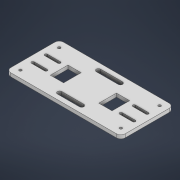
# Autodesk Inventor part: Top
Saved by Autodesk Inventor 2022.1 (Build 261234000, 234)
## iProperties
Created: 2021-10-08
Part Number: Top
Material: Generic
Document SubType Name: Modeling
Designer: Santiago Martínez
Mass: 26.6109 g
Surface Area: 166.584 cm^2
Volume: 26.6109 cm^3
Density: 1 g/cm^3
Appearance: Default
Author: Santiago Martínez
Autodesk Inventor part; units mm, degrees
ref_plane "YZ Plane" through (0, 0, 0) normal (1, 0, 0) x (0, 1, 0)
ref_plane "XZ Plane" through (0, 0, 0) normal (0, 1, 0) x (-1, 0, 0)
ref_plane "XY Plane" through (0, 0, 0) normal (0, 0, 1) x (1, 0, 0)
sketch "Motor Support" plane through (0, 0, 0) normal (1, 0, 0) x (0, 1, 0)
  circle A0 centre (0, 0) radius 11.25
  line L0 (-12.5, -22.5) -> (22.5, -22.5)
  line L1 (22.5, -22.5) -> (22.5, 22.5)
  line L2 (22.5, 22.5) -> (-12.5, 22.5)
  line L3 (-22.5, 12.5) -> (-22.5, -12.5)
  arc A1 (-12.5, 22.5) -> (-22.5, 12.5) centre (-12.5, 12.5) ccw
  arc A2 (-22.5, -12.5) -> (-12.5, -22.5) centre (-12.5, -12.5) ccw
  circle A3 centre (15.5, 15.5) radius 1.5
  circle A4 centre (15.5, -15.5) radius 1.5
  circle A5 centre (-15.5, 15.5) radius 1.5
  circle A6 centre (-15.5, -15.5) radius 1.5
  point P0 (-22.5, 22.5)
  point P1 (22.5, 0)
  dimension "d0" = 22.5
  dimension "d1" = 45
  dimension "d2" = 45
  dimension "d3" = 10
  dimension "d4" = 22.5
  dimension "d5" = 3
  dimension "d6" = 3
  dimension "d7" = 3
  dimension "d8" = 3
  dimension "d9" = 31
  dimension "d10" = 31
  dimension "d11" = 15.5
  dimension "d12" = 15.5
  constraints: 8 end point, 7 centre point, 4 point on circle, 4 tangent, 3 horizontal alignment, 2 parallel, 2 point on line, 2 vertical alignment, 1 coincident, 1 equal radius, 1 horizontal, 1 midpoint, 1 perpendicular
  measures "d0" diameter of A0
  measures "d1" distance of point (-22.5, 22.5) L1.end
  measures "d2" distance of L1.end L0.end
  measures "d3" radius of A1
  measures "d4" distance from line of L1 point (0, 0)
  measures "d5" diameter of A3
  measures "d6" diameter of A4
  measures "d7" diameter of A5
  measures "d8" diameter of A6
  measures "d9" distance of A4.centre A3.centre
  measures "d10" distance of A5.centre A3.centre
  measures "d11" horizontal distance of A3.centre point (0, 0)
  measures "d12" horizontal distance of A3.centre point (0, 0)
extrude "Motor Support E" add sketch "Motor Support" along normal blind 4
sketch "Base" plane through (0, 22.5, 22.5) normal (0, 1, 0) x (1, 0, 0)
  line L0 (0, 45) -> (0, 0) projected
  line L1 (0, 0) -> (4, 0) projected
  line L2 (4, 45) -> (4, 0) projected
  line L3 (0, 45) -> (4, 45) projected
  line L4 (4, -7.5) -> (-61, -7.5)
  line L5 (-61, -7.5) -> (-61, 52.5)
  line L6 (-61, 52.5) -> (4, 52.5)
  line L7 (4, 52.5) -> (4, -7.5)
  line L8 (-41, 32.5) -> (-26, 32.5)
  line L9 (-26, 32.5) -> (-26, 12.5)
  line L10 (-26, 12.5) -> (-41, 12.5)
  line L11 (-41, 12.5) -> (-41, 32.5)
  point P0 (0, 22.5)
  point P1 (4, 22.5)
  point P2 (-26, 22.5)
  point P3 (0, 22.5)
  dimension "d15" = 65
  dimension "d16" = 60
  dimension "d19" = 15
  dimension "d20" = 20
  dimension "d21" = 26
  constraints: 16 end point, 4 midpoint, 4 parallel, 2 horizontal, 2 perpendicular, 1 horizontal alignment
  measures "d15" distance of L5.end L6.end
  measures "d16" distance of L4.end L5.end
  measures "d19" distance of L9.end L10.end
  measures "d20" distance of L8.end L9.end
  measures "d21" distance between parallel lines of L0 L9
extrude "Base E" add sketch "Base" along normal blind 4
ref_plane "Mid Plane" through (-61, 26.5, 30) normal (-1, 0, 0) x (0, 0, 1)
mirror "Mirror Base" about plane through (-61, 26.5, 30) normal (-1, 0, 0)
fillet "Fillet1" radius 5 4 edges at (4, 24.5, 30) (4, 24.5, -30) (-126, 24.5, 30) (-126, 24.5, -30)
sketch "Base Hole Pattern" plane through (0, 26.5, 22.5) normal (0, 1, 0) x (1, 0, 0)
  circle A0 centre (-4, 0.5) radius 1.5
  circle A1 centre (-118, 44.5) radius 1.5
  circle A2 centre (-118, 0.5) radius 1.5
  circle A3 centre (-4, 44.5) radius 1.5
  arc A4 (-121, 52.5) -> (-126, 47.5) centre (-121, 47.5) ccw projected
  line L0 (-126, -2.5) -> (-126, 47.5) projected
  arc A5 (-126, -2.5) -> (-121, -7.5) centre (-121, -2.5) ccw projected
  line L1 (-1, -7.5) -> (-121, -7.5) projected
  arc A6 (-1, -7.5) -> (4, -2.5) centre (-1, -2.5) ccw projected
  line L2 (4, -2.5) -> (4, 47.5) projected
  arc A7 (4, 47.5) -> (-1, 52.5) centre (-1, 47.5) ccw projected
  line L3 (-1, 52.5) -> (-121, 52.5) projected
  line L4 (-81, 32.5) -> (-96, 32.5) projected
  line L5 (-81, 12.5) -> (-81, 32.5) projected
  line L6 (-96, 12.5) -> (-81, 12.5) projected
  line L7 (-96, 32.5) -> (-96, 12.5) projected
  line L8 (-41, 32.5) -> (-26, 32.5) projected
  line L9 (-26, 32.5) -> (-26, 12.5) projected
  line L10 (-26, 12.5) -> (-41, 12.5) projected
  line L11 (-41, 12.5) -> (-41, 32.5) projected
  line L12 (-73.5, 44.5) -> (-48.5, 44.5) construction
  line L13 (-73.5, 42) -> (-48.5, 42)
  line L14 (-48.5, 47) -> (-73.5, 47)
  arc A8 (-73.5, 47) -> (-73.5, 42) centre (-73.5, 44.5) ccw
  arc A9 (-48.5, 42) -> (-48.5, 47) centre (-48.5, 44.5) ccw
  line L15 (-73.5, 0.5) -> (-48.5, 0.5) construction
  line L16 (-73.5, -2) -> (-48.5, -2)
  line L17 (-48.5, 3) -> (-73.5, 3)
  arc A10 (-73.5, 3) -> (-73.5, -2) centre (-73.5, 0.5) ccw
  arc A11 (-48.5, -2) -> (-48.5, 3) centre (-48.5, 0.5) ccw
  line L18 (-118.5, 30) -> (-103.5, 30) construction
  line L19 (-118.5, 28.5) -> (-103.5, 28.5)
  line L20 (-103.5, 31.5) -> (-118.5, 31.5)
  arc A12 (-118.5, 31.5) -> (-118.5, 28.5) centre (-118.5, 30) ccw
  arc A13 (-103.5, 28.5) -> (-103.5, 31.5) centre (-103.5, 30) ccw
  line L21 (-118.5, 15) -> (-103.5, 15) construction
  line L22 (-118.5, 13.5) -> (-103.5, 13.5)
  line L23 (-103.5, 16.5) -> (-118.5, 16.5)
  arc A14 (-118.5, 16.5) -> (-118.5, 13.5) centre (-118.5, 15) ccw
  arc A15 (-103.5, 13.5) -> (-103.5, 16.5) centre (-103.5, 15) ccw
  line L24 (-18.5, 30) -> (-3.5, 30) construction
  line L25 (-18.5, 28.5) -> (-3.5, 28.5)
  line L26 (-3.5, 31.5) -> (-18.5, 31.5)
  arc A16 (-18.5, 31.5) -> (-18.5, 28.5) centre (-18.5, 30) ccw
  arc A17 (-3.5, 28.5) -> (-3.5, 31.5) centre (-3.5, 30) ccw
  line L27 (-18.5, 15) -> (-3.5, 15) construction
  line L28 (-18.5, 13.5) -> (-3.5, 13.5)
  line L29 (-3.5, 16.5) -> (-18.5, 16.5)
  arc A18 (-18.5, 16.5) -> (-18.5, 13.5) centre (-18.5, 15) ccw
  arc A19 (-3.5, 13.5) -> (-3.5, 16.5) centre (-3.5, 15) ccw
  point P0 (-61, 44.5)
  point P1 (-61, 52.5)
  point P2 (-61, 0.5)
  point P3 (-111, 30)
  point P4 (-111, 15)
  point P5 (-11, 30)
  point P6 (-11, 15)
  dimension "d29" = 3
  dimension "d30" = 3
  dimension "d33" = 3
  dimension "d34" = 3
  dimension "d35" = 8
  dimension "d36" = 8
  dimension "d37" = 8
  dimension "d38" = 8
  dimension "d43" = 25
  dimension "d44" = 5
  dimension "d45" = 25
  dimension "d46" = 2.5
  dimension "d47" = 15
  dimension "d48" = 3
  dimension "d49" = 15
  dimension "d50" = 3
  dimension "d51" = 15
  dimension "d52" = 15
  dimension "d53" = 22.5
  dimension "d56" = 15
  dimension "d57" = 3
  dimension "d58" = 15
  dimension "d59" = 3
  dimension "d60" = 15
  dimension "d61" = 22.5
  dimension "d62" = 15
  constraints: 48 end point, 24 point on circle, 24 tangent, 16 centre point, 7 midpoint, 7 parallel, 6 vertical alignment, 5 horizontal, 4 horizontal alignment
  measures "d29" diameter of A0
  measures "d30" diameter of A1
  measures "d33" diameter of A2
  measures "d34" diameter of A3
  measures "d35" distance from line of L3 A1.centre
  measures "d36" distance from line of L0 A1.centre
  measures "d37" distance from line of L2 A3.centre
  measures "d38" distance from line of L1 A0.centre
  measures "d43" distance of L12.start L12.end
  measures "d44" diameter of A9
  measures "d45" distance of L15.start L15.end
  measures "d46" radius of A11
  measures "d47" distance of L18.start L18.end
  measures "d48" diameter of A13
  measures "d49" distance of L21.start L21.end
  measures "d50" diameter of A15
  measures "d51" distance from line of L0 point (-111, 30)
  measures "d52" distance of point (-111, 30) point (-111, 15)
  measures "d53" distance from line of L3 point (-111, 30)
  measures "d56" distance of L24.start L24.end
  measures "d57" diameter of A17
  measures "d58" distance of L27.start L27.end
  measures "d59" diameter of A19
  measures "d60" distance of point (-11, 15) point (-11, 30)
  measures "d61" distance from line of L3 point (-11, 30)
  measures "d62" distance from line of L2 point (-11, 30)
extrude "Spacer Holes" cut sketch "Base Hole Pattern" against normal blind 10 contours A0 | A1 | A2 | A3
extrude "Base Slots" cut sketch "Base Hole Pattern" against normal blind 10 contours A8 L14 A9 L13 | A10 L17 A11 L16 | A12 L20 A13 L19 | A14 L23 A15 L22 | A16 L26 A17 L25 | A18 L29 A19 L28
sketch "Sketch6" plane through (0, -22.5, -12.5) normal (0, -1, 0) x (1, 0, 0)
  line L0 (11.3171, -23.408) -> (-133.75, -23.408)
  line L1 (-133.75, -23.408) -> (-133.75, 52.8884)
  line L2 (-133.75, 52.8884) -> (11.3171, 52.8884)
  line L3 (11.3171, 52.8884) -> (11.3171, -23.408)
  point P0 (0, 12.5)
  constraints: 8 end point, 2 parallel, 1 horizontal, 1 perpendicular
extrude "Remove Motor Support" cut sketch "Sketch6" against normal up to surface (45 mm away)
equation "\"d6\" = d5"
equation "\"d7\" = d5"
equation "\"d8\" = d5"
equation "\"d30\" = d29"
equation "\"d33\" = d29"
equation "\"d34\" = d29"
equation "\"d36\" = d35"
equation "\"d37\" = d35"
equation "\"d38\" = d35"
equation "\"d45\" = d43"
equation "\"d46\" = 0.5 * d44"
equation "\"d49\" = d47"
equation "\"d50\" = d48"
equation "\"d56\" = d47"
equation "\"d57\" = d48"
equation "\"d58\" = d47"
equation "\"d59\" = d48"
equation "\"d60\" = d52"
equation "\"d61\" = d53"
equation "\"d62\" = d51"
body "Solid1"
